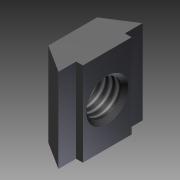
# Autodesk Inventor part: HNTT5-5_1
Saved by Autodesk Inventor 2011 SP1 (Build 150282100, 282)
## iProperties
Created: 2015-02-01
Part Number: HNTT5-5_1
Catalog Web Link: www.cadenas.de
Description: HNTTBS, HNTT, HNTTSN, HNTTSS_1-Pre-Assembly Fitting Nuts for Aluminum Frames_1
Vendor: MISUMI
Document SubType Name: Modeling
Designer: psAdmin
Manufacturer: MISUMI
Mass: 0.249463 g
Surface Area: 3.33953 cm^2
Volume: 0.249463 cm^3
Density: 1 g/cm^3
Category: PARTsolutions
Company: MISUMI
Title: HNTT5-5_1
Author: Cadenas PARTsolutions
Comments: Pre-Assembly Fitting Nuts for Aluminum Frames_1
PSOL_IDENT_0: {\\10.0.0.236\data_v8\23d-libs\misumi\metric\38_al_extrusions_blackets\nuts\hnttbs_1.prj},189 {VTYP=
PSOL_IDENT_1: 3D},{NB=HNTT5-5_1},{LINA=HNTT5-5_1},{NN=HNTTBS, HNTT, HNTTSN, HNTTSS_1},{DATE=19.11.2014 02:34:08},{
PSOL_IDENT_2: GEOMDATE=17.09.2009 00:00:00},{VERSION=},{LINEID=20},{LINESUBID=-1},{WBVAR=MAT,M}  {NB=HNTT5-5_1},{L
PSOL_IDENT_3: INA=HNTT5-5_1},{KT=DUMMY},{PN=HNTT5-5},{TP=HNTT},{MAT=1010 Steel (or Equivalent)},{ST=Trivalent Chro
PSOL_IDENT_4: mate},{NO=5},{M=5},{CFS=HFS5},{CFSW=6},{CFT=20, 40 sq.},{MATT='3','4','5'},{A=5.8},{B=10.0},{D=0.0},
PSOL_IDENT_5: {E=3.3},{T=4.1},{L=10},{MMIN=4.134},{MMAX=5},{TT=6.8},{MATALG='304 Stainless Steel','304 Stainless S
PSOL_IDENT_6: teel','1010 Steel (or Equivalent)','1010 Steel (or Equivalent)','316 Stainless Steel (or Equivalent)'
PSOL_IDENT_7: ,'316 Stainless Steel (or Equivalent)','303 Stainless Steel','303 Stainless Steel'},{X=0.7},{D11=6}
SUPPLIER: MISUMI
ARTICLENO: HNTT5-5_1
BOMINFO: HNTT5-5_1
CREATOR: CADENAS GmbH
Autodesk Inventor part; units mm, degrees
sketch "Sketch_4" plane through (0, 0, 0) normal (0, 0, 1) x (1, 0, 0)
  line L0 (-4.1, 2.9) -> (-4.1, -2.9)
  line L1 (-4.1, -2.9) -> (-0.8, -5)
  line L2 (-0.8, -5) -> (-0.8, -2.9)
  line L3 (-0.8, -2.9) -> (0, -2.9)
  line L4 (0, -2.9) -> (0, 2.9)
  line L5 (0, 2.9) -> (-0.8, 2.9)
  line L6 (-0.8, 2.9) -> (-0.8, 5)
  line L7 (-0.8, 5) -> (-4.1, 2.9)
  constraints: 16 end point
extrude "Extrusion1" add sketch "Sketch_4" along normal mid plane 10
sketch "Sketch_5" plane through (0, 0, 0) normal (0, 0, 1) x (1, 0, 0)
  line L0 (0, 0) -> (-4.1, 0)
  line L1 (-4.1, 0) -> (-4.1, 2.5)
  line L2 (-4.1, 2.5) -> (-3.667, 2.067)
  line L3 (-3.667, 2.067) -> (-0.433, 2.067)
  line L4 (-0.433, 2.067) -> (0, 2.5)
  line L5 (0, 2.5) -> (0, 0)
  line L6 (0, 0) -> (-4.1, 0)
  constraints: 14 end point
revolve "Revolution1" cut sketch "Sketch_5" angle 360 about axis through (0, 0, 0) along (1, 0, 0)
thread "Thread1" size "M5x0.8" class "6H" standard "ISO Metric profile" full length
ref_plane "nut_XY" through (0, 0, 0) normal (1, 0, 0) x (0, 0, -1)
ref_plane "nut_YZ" through (0, 0, 0) normal (0, 0, -1) x (0, 1, 0)
ref_plane "nut_ZX" through (0, 0, 0) normal (0, 1, 0) x (1, 0, 0)
ref_plane "to_bolt_XY" through (-4.1, 0, 0) normal (1, 0, 0) x (0, 0, -1)
ref_plane "to_bolt_YZ" through (-4.1, 0, 0) normal (0, 0, -1) x (0, 1, 0)
ref_plane "to_bolt_ZX" through (-4.1, 0, 0) normal (0, 1, 0) x (1, 0, 0)
ref_plane "to_frames_XY" through (-0.8, 0, 0) normal (1, 0, 0) x (0, 0, -1)
ref_plane "to_frames_YZ" through (-0.8, 0, 0) normal (0, 0, -1) x (0, 1, 0)
ref_plane "to_frames_ZX" through (-0.8, 0, 0) normal (0, 1, 0) x (1, 0, 0)
body "Solid1"
